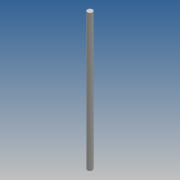
# Autodesk Inventor part: Eje guia
Saved by Autodesk Inventor 2016 (Build 200138000, 138)
## iProperties
Created: 2016-05-25
Part Number: Eje guia
Material: Generic
Document SubType Name: Modeling
Designer: Familia
Density: 1 g/cm^3
Appearance: Default
Mass: 1.3823 g
Surface Area: 14.0743 cm^2
Volume: 1.3823 cm^3
Author: Familia
Autodesk Inventor part; units mm, degrees
ref_plane "YZ Plane" through (0, 0, 0) normal (1, 0, 0) x (0, 1, 0)
ref_plane "XZ Plane" through (0, 0, 0) normal (0, 1, 0) x (-1, 0, 0)
ref_plane "XY Plane" through (0, 0, 0) normal (0, 0, 1) x (1, 0, 0)
sketch "Sketch1" plane through (0, 0, 0) normal (0, 1, 0) x (-1, 0, 0)
  line L0 (0, 0) -> (0, 110)
  line L1 (0, 110) -> (2, 110)
  line L2 (2, 110) -> (2, 0)
  line L3 (2, 0) -> (0, 0)
  line L4 (0, 0) -> (0, -3.3333)
  dimension "d0" = 4
  dimension "d1" = 110
  constraints: 10 end point, 2 perpendicular, 2 vertical, 1 parallel
  measures "d0" diameter of L2 L4
  measures "d1" distance between parallel lines of L1 L3
revolve "Revolution1" add sketch "Sketch1" angle 360 about axis through (0, 0, 0) along (0, 0, -1)
body "Solid1"
